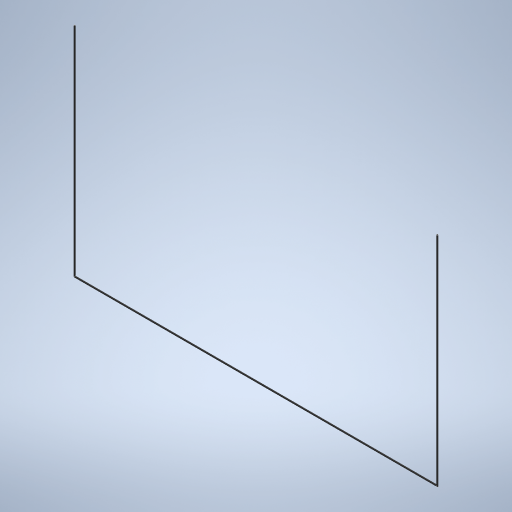
# Autodesk Inventor part: Gummidichtung
Saved by Autodesk Inventor 2024 (Build 280153000, 153)
## iProperties
Created: 2024-03-12
Part Number: Gummidichtung
Material: Gummi
Document SubType Name: Modeling
Designer: haniv
Density: 0.93 g/cm^3
Appearance: Gummi - Schwarz
Author: haniv
Autodesk Inventor part; units mm, degrees
ref_plane "YZ Plane" through (0, 0, 0) normal (1, 0, 0) x (0, 1, 0)
ref_plane "XZ Plane" through (0, 0, 0) normal (0, 1, 0) x (-1, 0, 0)
ref_plane "XY Plane" through (0, 0, 0) normal (0, 0, 1) x (1, 0, 0)
sketch "Skizze1" plane through (0, 0, 0) normal (0, 1, 0) x (-1, 0, 0)
  line L0 (-507, 0) -> (-507, -608)
  line L1 (-507, -608) -> (507, -608)
  line L2 (507, -608) -> (507, 0)
  circle A0 centre (504.5, -605.5) radius 2.5
  circle A1 centre (-504.5, -605.5) radius 2.5
  point P0 (0, 0)
  point P1 (0, 304)
  point P2 (0, -608)
  dimension "d0" = 1014
  dimension "d1" = 608
  dimension "d2" = 5
  constraints: 6 end point, 4 tangent, 2 centre point, 2 horizontal alignment, 2 vertical alignment, 1 equal radius, 1 midpoint, 1 parallel, 1 perpendicular, 1 vertical
  measures "d0" distance of L1.end L0.end
  measures "d1" distance of L1.end L2.end
  measures "d2" diameter of A0
sketch "Skizze2" plane through (0, 0, 0) normal (0, 0, 1) x (1, 0, 0)
  circle A0 centre (-507, 0) radius 2
  point P0 (0, 0)
  dimension "d3" = 4
  dimension "d4" = 507
  constraints: 1 centre point, 1 horizontal alignment
  measures "d3" diameter of A0
  measures "d4" distance of point (0, 0) A0.centre
sweep "Sweeping1" add profiles "Skizze2" path "Skizze1" path curves L2 L1 L0
